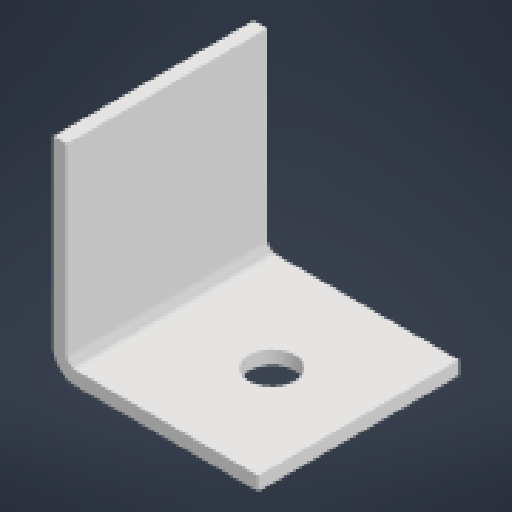
# Autodesk Inventor part: Angle_motor
Saved by Autodesk Inventor 2023.4 (Build 274418000, 418)
## iProperties
Created: 2025-09-23
Part Number: Angle_motor
Material: Generic
Document SubType Name: Modeling
Designer: Malthe Sennels
Density: 1 g/cm^3
Appearance: Default
Author: Malthe Sennels
Autodesk Inventor part; units mm, degrees
ref_plane "YZ Plane" through (0, 0, 0) normal (1, 0, 0) x (0, 1, 0)
ref_plane "XZ Plane" through (0, 0, 0) normal (0, 1, 0) x (-1, 0, 0)
ref_plane "XY Plane" through (0, 0, 0) normal (0, 0, 1) x (1, 0, 0)
sketch "Sketch1" plane through (0, 0, 0) normal (0, 0, 1) x (1, 0, 0)
  line L0 (19, 0) -> (-21, 0)
  line L1 (-26, 0) -> (-26, -3)
  line L2 (-26, -3) -> (19, -3)
  line L3 (19, -3) -> (19, 0)
  line L4 (-26, -3) -> (-23, -3)
  line L5 (-23, 2) -> (-23, 42)
  line L6 (-23, 42) -> (-26, 42)
  line L7 (-26, 42) -> (-26, -3)
  arc A0 (-23, 2) -> (-21, 0) centre (-21, 2) ccw
  arc A1 (-26, 2) -> (-21, -3) centre (-21, 2) ccw
  point P0 (0, 0)
  point P1 (19, -1.5)
  dimension "d0" = 45
  dimension "d1" = 19
  dimension "d2" = 45
  dimension "d3" = 3
  dimension "d4" = 3
  dimension "d5" = 2
  constraints: 16 end point, 5 point on line, 4 parallel, 4 point on circle, 3 tangent, 2 centre point, 2 horizontal, 2 perpendicular, 1 coincident, 1 midpoint
  measures "d0" distance of L2.end L1.end
  measures "d1" horizontal distance of point (19, -1.5) point (0, 0)
  measures "d2" distance of L5.end L4.end
  measures "d3" distance between parallel lines of L7 L5
  measures "d4" distance between parallel lines of L2 L0
  measures "d5" radius of A0
extrude "Extrusion1" add sketch "Sketch1" along normal mid plane 44 contours L3 L2 A1 L7 L6 L5 A0 L0
sketch "Sketch2" plane through (-21, -3, 22) normal (0, -1, 0) x (1, 0, 0)
  circle A0 centre (21, -22) radius 5
  dimension "d8" = 10
  constraints: 1 centre point, 1 coincident
  measures "d8" diameter of A0
extrude "Extrusion2" cut sketch "Sketch2" against normal through all
sketch "Sketch3" plane through (-21, -3, 22) normal (0, -1, 0) x (1, 0, 0)
  point P0 (21, -22)
sketch "Sketch4" plane through (-21, -3, 22) normal (0, -1, 0) x (1, 0, 0)
  line L0 (28.25, -14.75) -> (13.75, -14.75) construction
  line L1 (13.75, -14.75) -> (13.75, -29.25) construction
  line L2 (13.75, -29.25) -> (28.25, -29.25) construction
  line L3 (28.25, -29.25) -> (28.25, -14.75) construction
  line L4 (28.25, -14.75) -> (13.75, -29.25) construction
  line L5 (13.75, -14.75) -> (28.25, -29.25) construction
  circle A0 centre (28.25, -29.25) radius 1.75
  circle A1 centre (13.75, -29.25) radius 1.75
  circle A2 centre (13.75, -14.75) radius 1.75
  circle A3 centre (28.25, -14.75) radius 1.75
  point P0 (21, -22)
  dimension "d11" = 14.5
  dimension "d12" = 14.5
  dimension "d13" = 3.5
  dimension "d14" = 3.5
  dimension "d15" = 3.5
  dimension "d16" = 3.5
  constraints: 12 end point, 4 centre point, 3 coincident, 2 midpoint, 2 parallel, 1 horizontal, 1 perpendicular, 1 point on line
  measures "d11" distance of L2.end L1.end
  measures "d12" distance of L1.end L0.end
  measures "d13" diameter of A0
  measures "d14" diameter of A1
  measures "d15" diameter of A2
  measures "d16" diameter of A3
extrude "Extrusion3" cut sketch "Sketch4" against normal up to surface (3 mm away)
equation "\"d14\" = d13"
equation "\"d15\" = d13"
equation "\"d16\" = d13"
body "Solid1"
